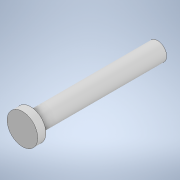
# Autodesk Inventor part: CilindroHidraulico_2
Saved by Autodesk Inventor 2021 (Build 250183000, 183)
## iProperties
Created: 2021-07-12
Part Number: CilindroHidraulico_2
Material: Generic
Document SubType Name: Modeling
Designer: Nelson
Density: 1 g/cm^3
Appearance: Default
Author: Nelson
Autodesk Inventor part; units mm, degrees
ref_plane "YZ Plane" through (0, 0, 0) normal (1, 0, 0) x (0, 1, 0)
ref_plane "XZ Plane" through (0, 0, 0) normal (0, 1, 0) x (-1, 0, 0)
ref_plane "XY Plane" through (0, 0, 0) normal (0, 0, 1) x (1, 0, 0)
sketch "Sketch3" plane through (0, 0, 0) normal (1, 0, 0) x (0, 1, 0)
  line L0 (0, 0) -> (75, 0)
  line L1 (0, 0) -> (0, -40)
  line L2 (0, -40) -> (30.5, -40)
  line L3 (30.5, -40) -> (30.5, -662)
  line L4 (75, 0) -> (75, -662)
  line L5 (75, -662) -> (30.5, -662)
  dimension "d3" = 75
  dimension "d4" = 40
  dimension "d6" = 622
  dimension "d8" = 44.5
  constraints: 12 end point, 3 vertical, 2 horizontal, 1 perpendicular
  measures "d3" distance of L0.start L0.end
  measures "d4" distance of L0.start L1.end
  measures "d6" distance of L2.end L3.end
  measures "d8" distance of L4.end L3.end
revolve "Revolution1" add sketch "Sketch3" angle 360 about axis through (0, 75, 0) along (0, 0, -1)
body "Solid1"
